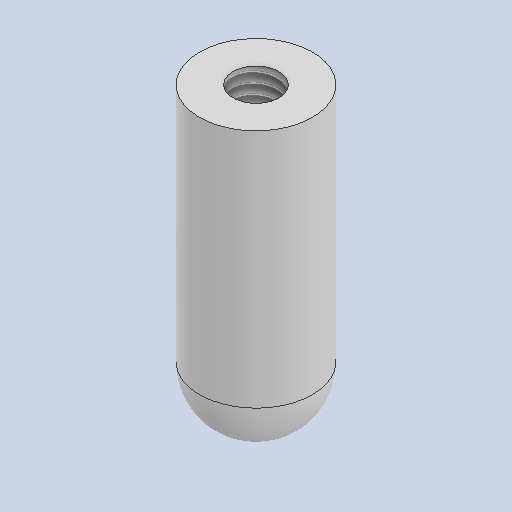
# Autodesk Inventor part: Dedo-02
Saved by Autodesk Inventor 2026 (Build 300175050, 175E)
## iProperties
Created: 2025-09-19
Part Number: Dedo-02
Material: Genérico
Document SubType Name: Modeling
Designer: Kedson Neves
Density: 1 g/cm^3
Appearance: Padrão
Author: Kedson Neves
Autodesk Inventor part; units mm, degrees
ref_plane "YZ Plane" through (0, 0, 0) normal (1, 0, 0) x (0, 1, 0)
ref_plane "XZ Plane" through (0, 0, 0) normal (0, 1, 0) x (-1, 0, 0)
ref_plane "XY Plane" through (0, 0, 0) normal (0, 0, 1) x (1, 0, 0)
sketch "Esboço1" plane through (0, 0, 0) normal (0, 1, 0) x (-1, 0, 0)
  circle A0 centre (0, 0) radius 4
  dimension "d0" = 8
  constraints: 1 centre point, 1 coincident
  measures "d0" diameter of A0
extrude "Extrusão1" add sketch "Esboço1" along normal blind 21
fillet "Arredondamento1" radius 4 1 edges at (4, 0, 0)
sketch "Esboço2" plane through (0, 21, 0) normal (0, 1, 0) x (1, 0, 0)
  point P0 (0, 0)
  point P1 (0, 0)
  constraints: 1 coincident
hole "Furo1" at (0, 21, 0) direction (0, -1, 0) diameter 3.242 depth 10 thread size "M4x0.7" class "6H" standard "ISO Metric profile"
